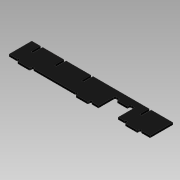
# Autodesk Inventor part: AK-C-C39-Separator
Saved by Autodesk Inventor 2016 (Build 200138000, 138)
## iProperties
Created: 2016-04-01
Part Number: AK-C-C39-Separator
Material: Generic
Document SubType Name: Modeling
Designer: admin
Density: 1 g/cm^3
Appearance: Glossy - Black
Mass: 3.01223 g
Surface Area: 43.5376 cm^2
Volume: 3.01223 cm^3
Author: admin
Autodesk Inventor part; units mm, degrees
ref_plane "YZ Plane" through (0, 0, 0) normal (1, 0, 0) x (0, 1, 0)
ref_plane "XZ Plane" through (0, 0, 0) normal (0, 1, 0) x (-1, 0, 0)
ref_plane "XY Plane" through (0, 0, 0) normal (0, 0, 1) x (1, 0, 0)
sketch "Sketch1" plane through (0, 0, 0) normal (0, 0, 1) x (1, 0, 0)
  line L0 (-57, -9.2) -> (-57, 9.2)
  line L1 (-57, 9.2) -> (-50, 9.2)
  line L2 (-50, 9.2) -> (-50, 2.2)
  line L3 (-48.25, 2.2) -> (-48.25, 9.2)
  line L4 (-48.25, 9.2) -> (-31, 9.2)
  line L5 (-31, 9.2) -> (-31, 2.2)
  line L6 (-29.25, 2.2) -> (-29.25, 9.2)
  line L7 (-29.25, 9.2) -> (-9.25, 9.2)
  line L8 (-9.25, 9.2) -> (-9.25, 2.2)
  line L9 (-7.5, 2.2) -> (-7.5, 9.2)
  line L10 (-7.5, 9.2) -> (37.75, 9.2)
  line L11 (37.75, 9.2) -> (37.75, 2.2)
  line L12 (39.5, 2.2) -> (39.5, 9.2)
  line L13 (39.5, 9.2) -> (57, 9.2)
  line L14 (57, 9.2) -> (57, -9.2)
  line L15 (57, -9.2) -> (50, -9.2)
  line L16 (48.25, -9.2) -> (48.25, -10.2)
  line L17 (47.75, -10.7) -> (38.75, -10.7)
  line L18 (38.25, -10.2) -> (38.25, -9.2)
  line L19 (8.25, -9.2) -> (8.25, -10.2)
  line L20 (7.75, -10.7) -> (-1.25, -10.7)
  line L21 (-1.75, -10.2) -> (-1.75, -9.2)
  line L22 (-3.5, -9.2) -> (-37, -9.2)
  line L23 (-38.75, -9.2) -> (-38.75, -10.2)
  line L24 (-39.25, -10.7) -> (-48.25, -10.7)
  line L25 (-48.75, -10.2) -> (-48.75, -9.2)
  line L26 (-50.5, -9.2) -> (-57, -9.2)
  arc A0 (-50, 2.2) -> (-48.25, 2.2) centre (-49.125, 2.2) ccw
  arc A1 (-31, 2.2) -> (-29.25, 2.2) centre (-30.125, 2.2) ccw
  arc A2 (-9.25, 2.2) -> (-7.5, 2.2) centre (-8.375, 2.2) ccw
  arc A3 (37.75, 2.2) -> (39.5, 2.2) centre (38.625, 2.2) ccw
  arc A4 (50, -9.2) -> (48.25, -9.2) centre (49.125, -9.2) ccw
  arc A5 (38.25, -9.2) -> (36.5, -9.2) centre (37.375, -9.2) ccw
  arc A6 (10, -9.2) -> (8.25, -9.2) centre (9.125, -9.2) ccw
  arc A7 (-1.75, -9.2) -> (-3.5, -9.2) centre (-2.625, -9.2) ccw
  arc A8 (-37, -9.2) -> (-38.75, -9.2) centre (-37.875, -9.2) ccw
  arc A9 (-48.75, -9.2) -> (-50.5, -9.2) centre (-49.625, -9.2) ccw
  line L27 (0, 7.1627) -> (0, -7.1627) construction
  line L28 (-57.5, 4.3673) -> (-57.5, -4.382) construction
  line L29 (57.5, 7.0555) -> (57.5, -5.2201) construction
  line L30 (-48.75, -10.2) -> (-48.25, -10.7)
  line L31 (-39.25, -10.7) -> (-38.75, -10.2)
  line L32 (-1.75, -10.2) -> (-1.25, -10.7)
  line L33 (7.75, -10.7) -> (8.25, -10.2)
  line L34 (38.25, -10.2) -> (38.75, -10.7)
  line L35 (47.75, -10.7) -> (48.25, -10.2)
  line L36 (15.75, 2.14) -> (30.75, 2.14) construction
  line L37 (30.75, 2.14) -> (30.75, -9.2) construction
  line L38 (15.75, -9.2) -> (15.75, 2.14) construction
  line L39 (15.25, -9.2) -> (15.25, 3.34)
  line L40 (31.25, 3.34) -> (31.25, -9.2)
  line L41 (16.75, 2.14) -> (16.75, 4.34) construction
  line L42 (16.75, 4.34) -> (17.75, 4.34) construction
  line L43 (17.75, 4.34) -> (17.75, 2.14) construction
  line L44 (28.75, 2.14) -> (28.75, 4.34) construction
  line L45 (28.75, 4.34) -> (29.75, 4.34) construction
  line L46 (29.75, 4.34) -> (29.75, 2.14) construction
  line L47 (19.25, 2.14) -> (27.25, 2.14)
  line L48 (23.25, -1.4722) -> (23.25, -5.1824) construction
  line L49 (17.25, 3.637) -> (17.25, 2.3773) construction
  arc A10 (28.25, 4.34) -> (27.25, 3.34) centre (28.25, 3.34) ccw
  arc A11 (31.25, 3.34) -> (30.25, 4.34) centre (30.25, 3.34) ccw
  line L50 (19.25, 3.34) -> (19.25, 2.14)
  line L51 (27.25, 3.34) -> (27.25, 2.14)
  line L52 (10, -9.2) -> (15.25, -9.2)
  line L53 (31.25, -9.2) -> (36.5, -9.2)
  line L54 (15.75, -9.2) -> (30.75, -9.2) construction
  arc A12 (16.25, 4.34) -> (15.25, 3.34) centre (16.25, 3.34) ccw
  arc A13 (19.25, 3.34) -> (18.25, 4.34) centre (18.25, 3.34) ccw
  line L55 (16.25, 4.34) -> (18.25, 4.34)
  line L56 (29.25, 3.708) -> (29.25, 2.5772) construction
  line L57 (28.25, 4.34) -> (30.25, 4.34)
  point P0 (0, 0)
  point P1 (0, 0)
  point P2 (57, 0)
  dimension "d2" = 1.75
  dimension "d3" = 7
  dimension "d7" = 1.5
  dimension "d11" = 37
  dimension "d12" = 30
  dimension "d15" = 115
  dimension "d16" = 0.5
  dimension "d17" = 0.5
  dimension "d18" = 8.75
  dimension "d19" = 9.25
  dimension "d22" = 20
  dimension "d23" = 47
  dimension "d24" = 18.4
  dimension "d25" = 135
  dimension "d26" = 0.5
  dimension "d27" = 10
  dimension "d28" = 10
  dimension "d29" = 10
  dimension "d31" = 7
  dimension "d32" = 15
  dimension "d34" = 19
  dimension "d36" = 16
  dimension "d38" = 11.34
  dimension "d39" = 1
  dimension "d40" = 12
  dimension "d41" = 2.2
  constraints: 117 end point, 28 point on circle, 22 point on line, 21 tangent, 19 vertical, 16 perpendicular, 14 centre point, 12 equal radius, 9 collinear, 9 horizontal, 6 equal length, 6 horizontal alignment, 5 parallel, 2 midpoint, 1 coincident, 1 symmetric about line, 8 other
  measures "d2" diameter of A9
  measures "d3" distance from line of A0.centre L1
  measures "d7" distance between parallel lines of L22 L24
  measures "d11" distance between parallel lines of L21 L23
  measures "d12" distance between parallel lines of L18 L19
  measures "d15" distance between parallel lines of L29 L28
  measures "d16" distance between parallel lines of L28 L0
  measures "d17" distance between parallel lines of L29 L14
  measures "d18" distance between parallel lines of L25 L28
  measures "d19" distance between parallel lines of L29 L16
  measures "d22" distance between parallel lines of L8 L6
  measures "d23" distance between parallel lines of L11 L8
  measures "d24" distance between parallel lines of L15 L13
  measures "d25" angle of L24 L30
  measures "d26" distance from line of L25.start L24
  measures "d27" distance between parallel lines of L16 L18
  measures "d28" distance between parallel lines of L19 L21
  measures "d29" distance between parallel lines of L23 L25
  measures "d31" distance between parallel lines of L2 L0
  measures "d32" distance between parallel lines of L37 L38
  measures "d34" distance between parallel lines of L6 L3
  measures "d36" distance between parallel lines of L40 L39
  measures "d38" distance between parallel lines of L54 L36
  measures "d39" distance between parallel lines of L41 L43
  measures "d40" distance between parallel lines of L56 L49
  measures "d41" distance between parallel lines of L36 L42
extrude "Extrusion1" add sketch "Sketch1" along normal blind 1.6
body "Solid1"
